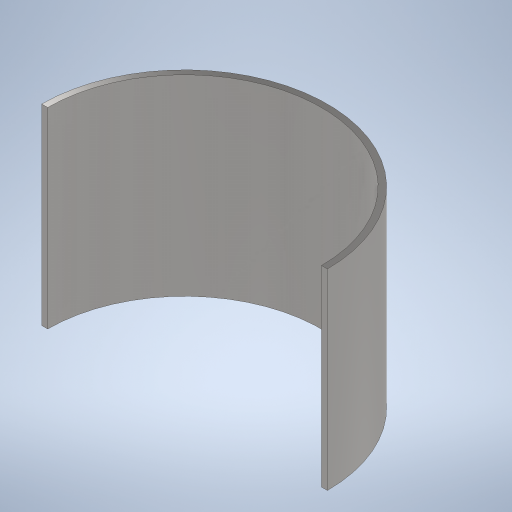
# Autodesk Inventor part: CollarTube
Saved by Autodesk Inventor 2024 (Build 280153000, 153)
## iProperties
Created: 2023-10-25
Part Number: CollarTube
Material: Stainless Steel
Document SubType Name: Modeling
Designer: schanen
Density: 8 g/cm^3
Appearance: Semi-Polished
Mass: 1013.35 g
Surface Area: 870.849 cm^2
Volume: 126.669 cm^3
Author: schanen
Autodesk Inventor part; units mm, degrees
ref_plane "YZ Plane" through (0, 0, 0) normal (1, 0, 0) x (0, 1, 0)
ref_plane "XZ Plane" through (0, 0, 0) normal (0, 1, 0) x (-1, 0, 0)
ref_plane "XY Plane" through (0, 0, 0) normal (0, 0, 1) x (1, 0, 0)
sketch "Sketch1" plane through (0, 0, 0) normal (0, 0, 1) x (1, 0, 0)
  line L0 (-68.5, 0) -> (-71.5, 0)
  line L1 (-71.5, 0) -> (-71.5, 96)
  line L2 (-71.5, 96) -> (-68.5, 96)
  line L3 (-68.5, 96) -> (-68.5, 0)
  line L4 (0, -19.2) -> (0, 115.2) projected
  point P0 (0, 0)
  dimension "d0" = 71.5
  dimension "d1" = 68.5
  dimension "d2" = 96
  dimension "d3" = 3
  constraints: 8 end point, 2 parallel, 1 horizontal, 1 horizontal alignment, 1 perpendicular
  measures "d0" distance from line of point (0, 0) L1
  measures "d1" distance from line of point (0, 0) L3
  measures "d2" distance of L0.end L1.end
  measures "d3" distance between parallel lines of L3 L1
revolve "Revolution1" add sketch "Sketch1" angle 360 about axis through (0, -10, 0) along (0, 1, 0)
sketch "Sketch2" plane through (0, 96, 0) normal (0, 1, 0) x (1, 0, 0)
  circle A0 centre (0, 0) radius 71.5 projected
  line L0 (-71.5, 0) -> (71.5, 0)
  line L1 (71.5, 0) -> (71.5, -71.5)
  line L2 (71.5, -71.5) -> (-71.5, -71.5)
  line L3 (-71.5, -71.5) -> (-71.5, 0)
  constraints: 8 end point, 2 parallel, 1 horizontal, 1 horizontal alignment, 1 perpendicular, 1 other
extrude "Extrusion1" cut sketch "Sketch2" against normal up to surface (96 mm away) contours L1 L2 A0 | A0 L0 | A0 L2 L3 picked at (-19.157, -31.4012)
body "Solid1"
